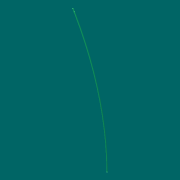
# Autodesk Inventor part: Long Fiber
Saved by Autodesk Inventor 2016 (Build 200138000, 138)
## iProperties
Created: 2015-08-14
Part Number: Long Fiber
Material: Glass
Document SubType Name: Modeling
Designer: Cosmic
Density: 2.18 g/cm^3
Appearance: Clear - Green 1
Author: Cosmic
Autodesk Inventor part; units mm, degrees
ref_plane "YZ Plane" through (0, 0, 0) normal (1, 0, 0) x (0, 1, 0)
ref_plane "XZ Plane" through (0, 0, 0) normal (0, 1, 0) x (-1, 0, 0)
ref_plane "XY Plane" through (0, 0, 0) normal (0, 0, 1) x (1, 0, 0)
sketch "Sketch1" plane through (0, 0, 0) normal (0, 0, 1) x (1, 0, 0)
  circle A0 centre (263.15, 0) radius 0.5
  line L0 (0, -0.7) -> (0, 0.7) projected
  point P0 (0, 0)
  dimension "d0" = 1
  dimension "d1" = 263.15
  dimension "d2" = 0
  constraints: 1 centre point
  measures "d0" diameter of A0
  measures "d1" distance of point (0, 0) A0.centre
  measures "d2" vertical distance of A0.centre point (0, 0)
revolve "Revolution1" add sketch "Sketch1" angle 30 about axis through (0, -10, 0) along (0, -1, 0)
sketch "Sketch2" plane through (227.8946, 0, 131.575) normal (-0.5, 0, 0.8660254) x (0.8660254, 0, 0.5)
  circle A0 centre (0, 0) radius 0.5 projected
  line L0 (-49.45, 0.5) -> (-49.45, -0.5) projected
  point P0 (-263.15, 0)
extrude "Extrusion1" add sketch "Sketch2" along normal blind 3
equation "\"d0\" = OpticalFiberDiameter"
equation "\"d3\" = LongFiberAngle"
equation "\"d4\" = ScintillatorEdgeClearence - MPPCDepth"
equation "\"OpticalFiberDiameter\" = 1"
equation "\"OpticalFiberClearence\" = 0.15"
equation "\"SmallTrackDiameter\" = 175"
equation "\"ScintillatorEdgeClearence\" = 3"
equation "\"ScintillatorWidth\" = 145"
equation "\"ScintillatorHeight\" = 145"
equation "\"ShallowTrackDepth\" = 1.3"
equation "\"MPPCClearence\" = 0.075"
equation "\"MPPCSensorClearence\" = 1.45"
equation "\"MPPCSensorOffsett\" = 2.105"
equation "\"MPPCWidth\" = 5.9"
equation "\"MPPCHeight\" = 6.55"
equation "\"FiberEdgeOffsett\" = 5"
equation "\"MPPCDepth\" = 0"
equation "\"LongFiberAngle\" = 30deg"
equation "\"ShortFiberAngle\" = 78deg"
equation "\"LoopLargeTrackRatio\" = 1.1"
equation "\"FiberSensorClerence\" = 0.5"
equation "\"MountingScrewDepth\" = 4"
body "Solid1"
